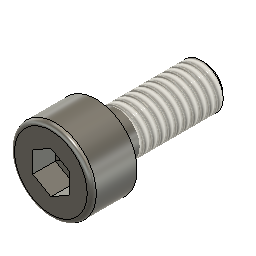
Spacemouse_3D_model (Autodesk Fusion 360 archive; units mm, degrees)
design "Broached Hexagon Socket Head Cap Screw ASME B18.3.1M - M2.5x0.45 x 6 Steel Grade 2 Plain"
description: Broached Hexagon Socket Head Cap Screw ASME B18.3.1M - M2.5x0.45 x 6
part number: BSHCS ASME B18.3.1M - M2.5x0.45 x 6 Steel Grade 2 Plain
Autodesk Fusion 360 part; units mm, degrees
sketch "Sketch1" plane through (0, 0, 0) normal (0, 1, 0) x (1, 0, 0)
  line L0 (-1.25, 0) -> (-1.25, 6)
  line L1 (-1.25, 6) -> (0, 6)
  line L2 (0, 6) -> (0, -2.5)
  line L3 (-1.25, 0) -> (-2.25, 0)
  line L4 (-2.25, 0) -> (-2.25, -2.5)
  line L5 (-2.25, -2.5) -> (0, -2.5)
  dimension "d101" = 6
  dimension "d102" = 2.5
  dimension "d109" = 4.5
  dimension "d110" = 2.5
  constraint perpendicular L0 L1
  constraint collinear origin L1.end L2.end
  constraint perpendicular L0 L3
  constraint coincident origin L3
  constraint vertical L2
  constraint coincident L2 L5.end
  constraint perpendicular L2 L5
  measures "d101" distance of origin L1
  measures "d102" distance of L3.end L5
revolve "Revolve1" add sketch "Sketch1" angle 360 about axis through (0, 0, -6) along (0, 0, 1)
ref_plane "WorkPlane1" through (0, 0, 2.5) normal (0, 0, 1) x (1, 0, 0)
sketch "Sketch6" plane through (0, 0, 2.5) normal (0, 0, 1) x (1, 0, 0)
  line L0 (0, -1.1547) -> (1, -0.5774)
  line L1 (1, -0.5774) -> (1, 0.5774)
  line L2 (1, 0.5774) -> (0, 1.1547)
  line L3 (0, 1.1547) -> (-1, 0.5774)
  line L4 (-1, 0.5774) -> (-1, -0.5774)
  line L5 (-1, -0.5774) -> (0, -1.1547)
  dimension "d111" = 2
  constraint vertical L1
  measures "d111" distance of L1 L4
extrude "Extrude1" cut sketch "Sketch6" against normal blind 1.25
extrude "Extrude2" cut 1 faces at (-0.3333, -0.1925, 1.25) along direction (0, 0, -1) blind 1.25 draft -85
thread "Thread3" "ANSI Metric M Profile 2.5 M2.5x0.45 M2.5x0.45 4g6g" major diameter 2.43 minor diameter 1.9295 pitch 0.45 angle 60 resizes the face on face at (-1.2438, 0.1245, -4) from (0, 0, -1.1761) to (0, 0, -6)
fillet "Fillet4" radius 0.25 1 edges at (-2.0977, 0.8136, 2.5)
sketch "Sketch7" plane through (0, 0, 0) normal (0, 1, 0) x (1, 0, 0)
  line L0 (-1.275, 6) -> (-1.275, 5.7239)
  line L1 (-1.275, 5.7239) -> (-0.9739, 6)
  line L2 (0, 6) -> (0, -2.5)
  line L3 (-1.275, 6) -> (0, 6)
  dimension "d104" = 0.9739
  dimension "d105" = 1.275
  dimension "d106" = 0.2761
  constraint coincident L2.start L3.end
  constraint perpendicular L2 L3
  constraint coincident L1.end L3
  constraint perpendicular L0 L3
  measures "d104" distance of L1.end L2
  measures "d105" distance of L0 L2.start
  measures "d106" distance of L0.end L3
revolve "Revolve3" cut sketch "Sketch7" angle 360 about axis through (0, 0, 1.75) along (0, 0, 1)
equation "adsk_nomlen = 6.000 mm"
equation "adsk_headh = 2.500 mm"
equation "adsk_headdia = 4.500 mm"
equation "adsk_nomdia = 2.500 mm"
equation "adsk_philwidth = 2.000 mm"
equation "d31 = -adsk_phildepth"
equation "adsk_phildepth = 1.250 mm"
equation "d71 = adsk_headh"
equation "d76 = -adsk_phildepth"
equation "adsk_thrlen = 4.8239475 mm"
equation "d86 = adsk_nomdia * 0.1"
equation "adsk_startlen = 0.2760525 mm"
equation "adsk_endpointdia = 1.947895 mm"
equation "d101 = adsk_nomlen"
equation "d102 = adsk_headh"
equation "d104 = adsk_endpointdia / 2"
equation "d105 = adsk_nomdia * 0.51"
equation "d106 = adsk_startlen"
equation "d108 = min(adsk_thrlen; adsk_nomlen - 0.001 mm)"
equation "d109 = adsk_headdia"
equation "d110 = adsk_nomdia"
equation "d111 = adsk_philwidth"

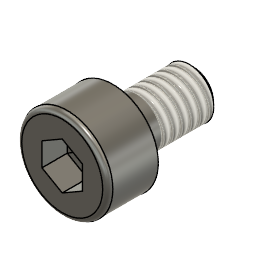
design "Vis percée à tête à six pans creux ASME B18.3.1M - M2.5x0.45 x 4 Acier de classe 2 Standard"
description: Vis percée à tête à six pans creux ASME B18.3.1M - M2.5x0.45 x 4
part number: BSHCS ASME B18.3.1M - M2.5x0.45 x 4 Acier de classe 2 Standard
Autodesk Fusion 360 part; units mm, degrees
sketch "Sketch1" plane through (0, 0, 0) normal (0, 1, 0) x (1, 0, 0)
  line L0 (-1.25, 0) -> (-1.25, 4)
  line L1 (-1.25, 4) -> (0, 4)
  line L2 (0, 4) -> (0, -2.5)
  line L3 (-1.25, 0) -> (-2.25, 0)
  line L4 (-2.25, 0) -> (-2.25, -2.5)
  line L5 (-2.25, -2.5) -> (0, -2.5)
  dimension "d101" = 4
  dimension "d102" = 2.5
  dimension "d109" = 4.5
  dimension "d110" = 2.5
  constraint perpendicular L0 L1
  constraint collinear origin L1.end L2.end
  constraint perpendicular L0 L3
  constraint coincident origin L3
  constraint vertical L2
  constraint coincident L2 L5.end
  constraint perpendicular L2 L5
  measures "d101" distance of origin L1
  measures "d102" distance of L3.end L5
revolve "Revolve1" add sketch "Sketch1" angle 360 about axis through (0, 0, -4) along (0, 0, 1)
ref_plane "WorkPlane1" through (0, 0, 2.5) normal (0, 0, 1) x (1, 0, 0)
sketch "Sketch6" plane through (0, 0, 2.5) normal (0, 0, 1) x (1, 0, 0)
  line L0 (0, -1.1547) -> (1, -0.5774)
  line L1 (1, -0.5774) -> (1, 0.5774)
  line L2 (1, 0.5774) -> (0, 1.1547)
  line L3 (0, 1.1547) -> (-1, 0.5774)
  line L4 (-1, 0.5774) -> (-1, -0.5774)
  line L5 (-1, -0.5774) -> (0, -1.1547)
  dimension "d111" = 2
  constraint vertical L1
  measures "d111" distance of L1 L4
extrude "Extrude1" cut sketch "Sketch6" against normal blind 1.25
extrude "Extrude2" cut 1 faces at (-0.3333, -0.1925, 1.25) along direction (0, 0, -1) blind 1.25 draft -85
thread "Thread3" "ANSI Metric M Profile 2.5 M2.5x0.45 M2.5x0.45 4g6g" major diameter 2.43 minor diameter 1.9295 pitch 0.45 angle 60 resizes the face on face at (-1.2484, 0.0623, -2.6667) from (0, 0, -1.1761) to (0, 0, -4)
fillet "Fillet4" radius 0.25 1 edges at (-2.0977, 0.8136, 2.5)
sketch "Sketch7" plane through (0, 0, 0) normal (0, 1, 0) x (1, 0, 0)
  line L0 (-1.275, 4) -> (-1.275, 3.7239)
  line L1 (-1.275, 3.7239) -> (-0.9739, 4)
  line L2 (0, 4) -> (0, -2.5)
  line L3 (-1.275, 4) -> (0, 4)
  dimension "d104" = 0.9739
  dimension "d105" = 1.275
  dimension "d106" = 0.2761
  constraint coincident L2.start L3.end
  constraint perpendicular L2 L3
  constraint coincident L1.end L3
  constraint perpendicular L0 L3
  measures "d104" distance of L1.end L2
  measures "d105" distance of L0 L2.start
  measures "d106" distance of L0.end L3
revolve "Revolve3" cut sketch "Sketch7" angle 360 about axis through (0, 0, 1.75) along (0, 0, 1)
equation "adsk_nomlen = 4.000 mm"
equation "adsk_headh = 2.500 mm"
equation "adsk_headdia = 4.500 mm"
equation "adsk_nomdia = 2.500 mm"
equation "adsk_philwidth = 2.000 mm"
equation "d31 = -adsk_phildepth"
equation "adsk_phildepth = 1.250 mm"
equation "d71 = adsk_headh"
equation "d76 = -adsk_phildepth"
equation "adsk_thrlen = 2.8239475 mm"
equation "d86 = adsk_nomdia * 0.1"
equation "adsk_startlen = 0.2760525 mm"
equation "adsk_endpointdia = 1.947895 mm"
equation "d101 = adsk_nomlen"
equation "d102 = adsk_headh"
equation "d104 = adsk_endpointdia / 2"
equation "d105 = adsk_nomdia * 0.51"
equation "d106 = adsk_startlen"
equation "d108 = min(adsk_thrlen; adsk_nomlen - 0.001 mm)"
equation "d109 = adsk_headdia"
equation "d110 = adsk_nomdia"
equation "d111 = adsk_philwidth"

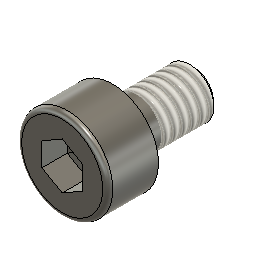
design "Broached Hexagon Socket Head Cap Screw ASME B18.3.1M - M2.5x0.45 x 4 Steel Grade 2 Plain"
description: Broached Hexagon Socket Head Cap Screw ASME B18.3.1M - M2.5x0.45 x 4
part number: BSHCS ASME B18.3.1M - M2.5x0.45 x 4 Steel Grade 2 Plain
Autodesk Fusion 360 part; units mm, degrees
sketch "Sketch1" plane through (0, 0, 0) normal (0, 1, 0) x (1, 0, 0)
  line L0 (-1.25, 0) -> (-1.25, 4)
  line L1 (-1.25, 4) -> (0, 4)
  line L2 (0, 4) -> (0, -2.5)
  line L3 (-1.25, 0) -> (-2.25, 0)
  line L4 (-2.25, 0) -> (-2.25, -2.5)
  line L5 (-2.25, -2.5) -> (0, -2.5)
  dimension "d101" = 4
  dimension "d102" = 2.5
  dimension "d109" = 4.5
  dimension "d110" = 2.5
  constraint perpendicular L0 L1
  constraint collinear origin L1.end L2.end
  constraint perpendicular L0 L3
  constraint coincident origin L3
  constraint vertical L2
  constraint coincident L2 L5.end
  constraint perpendicular L2 L5
  measures "d101" distance of origin L1
  measures "d102" distance of L3.end L5
revolve "Revolve1" add sketch "Sketch1" angle 360 about axis through (0, 0, -4) along (0, 0, 1)
ref_plane "WorkPlane1" through (0, 0, 2.5) normal (0, 0, 1) x (1, 0, 0)
sketch "Sketch6" plane through (0, 0, 2.5) normal (0, 0, 1) x (1, 0, 0)
  line L0 (0, -1.1547) -> (1, -0.5774)
  line L1 (1, -0.5774) -> (1, 0.5774)
  line L2 (1, 0.5774) -> (0, 1.1547)
  line L3 (0, 1.1547) -> (-1, 0.5774)
  line L4 (-1, 0.5774) -> (-1, -0.5774)
  line L5 (-1, -0.5774) -> (0, -1.1547)
  dimension "d111" = 2
  constraint vertical L1
  measures "d111" distance of L1 L4
extrude "Extrude1" cut sketch "Sketch6" against normal blind 1.25
extrude "Extrude2" cut 1 faces at (-0.3333, -0.1925, 1.25) along direction (0, 0, -1) blind 1.25 draft -85
thread "Thread3" "ANSI Metric M Profile 2.5 M2.5x0.45 M2.5x0.45 4g6g" major diameter 2.43 minor diameter 1.9295 pitch 0.45 angle 60 resizes the face on face at (-1.2484, 0.0623, -2.6667) from (0, 0, -1.1761) to (0, 0, -4)
fillet "Fillet4" radius 0.25 1 edges at (-2.0977, 0.8136, 2.5)
sketch "Sketch7" plane through (0, 0, 0) normal (0, 1, 0) x (1, 0, 0)
  line L0 (-1.275, 4) -> (-1.275, 3.7239)
  line L1 (-1.275, 3.7239) -> (-0.9739, 4)
  line L2 (0, 4) -> (0, -2.5)
  line L3 (-1.275, 4) -> (0, 4)
  dimension "d104" = 0.9739
  dimension "d105" = 1.275
  dimension "d106" = 0.2761
  constraint coincident L2.start L3.end
  constraint perpendicular L2 L3
  constraint coincident L1.end L3
  constraint perpendicular L0 L3
  measures "d104" distance of L1.end L2
  measures "d105" distance of L0 L2.start
  measures "d106" distance of L0.end L3
revolve "Revolve3" cut sketch "Sketch7" angle 360 about axis through (0, 0, 1.75) along (0, 0, 1)
equation "adsk_nomlen = 4.000 mm"
equation "adsk_headh = 2.500 mm"
equation "adsk_headdia = 4.500 mm"
equation "adsk_nomdia = 2.500 mm"
equation "adsk_philwidth = 2.000 mm"
equation "d31 = -adsk_phildepth"
equation "adsk_phildepth = 1.250 mm"
equation "d71 = adsk_headh"
equation "d76 = -adsk_phildepth"
equation "adsk_thrlen = 2.8239475 mm"
equation "d86 = adsk_nomdia * 0.1"
equation "adsk_startlen = 0.2760525 mm"
equation "adsk_endpointdia = 1.947895 mm"
equation "d101 = adsk_nomlen"
equation "d102 = adsk_headh"
equation "d104 = adsk_endpointdia / 2"
equation "d105 = adsk_nomdia * 0.51"
equation "d106 = adsk_startlen"
equation "d108 = min(adsk_thrlen; adsk_nomlen - 0.001 mm)"
equation "d109 = adsk_headdia"
equation "d110 = adsk_nomdia"
equation "d111 = adsk_philwidth"

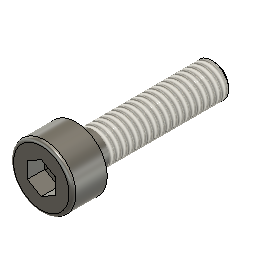
design "Broached Hexagon Socket Head Cap Screw ASME B18.3.1M - M2.5x0.45 x 10 Steel Grade 2 Plain"
description: Broached Hexagon Socket Head Cap Screw ASME B18.3.1M - M2.5x0.45 x 10
part number: BSHCS ASME B18.3.1M - M2.5x0.45 x 10 Steel Grade 2 Plain
Autodesk Fusion 360 part; units mm, degrees
sketch "Sketch1" plane through (0, 0, 0) normal (0, 1, 0) x (1, 0, 0)
  line L0 (-1.25, 0) -> (-1.25, 10)
  line L1 (-1.25, 10) -> (0, 10)
  line L2 (0, 10) -> (0, -2.5)
  line L3 (-1.25, 0) -> (-2.25, 0)
  line L4 (-2.25, 0) -> (-2.25, -2.5)
  line L5 (-2.25, -2.5) -> (0, -2.5)
  dimension "d101" = 10
  dimension "d102" = 2.5
  dimension "d109" = 4.5
  dimension "d110" = 2.5
  constraint perpendicular L0 L1
  constraint collinear origin L1.end L2.end
  constraint perpendicular L0 L3
  constraint coincident origin L3
  constraint vertical L2
  constraint coincident L2 L5.end
  constraint perpendicular L2 L5
  measures "d101" distance of origin L1
  measures "d102" distance of L3.end L5
revolve "Revolve1" add sketch "Sketch1" angle 360 about axis through (0, 0, -10) along (0, 0, 1)
ref_plane "WorkPlane1" through (0, 0, 2.5) normal (0, 0, 1) x (1, 0, 0)
sketch "Sketch6" plane through (0, 0, 2.5) normal (0, 0, 1) x (1, 0, 0)
  line L0 (0, -1.1547) -> (1, -0.5774)
  line L1 (1, -0.5774) -> (1, 0.5774)
  line L2 (1, 0.5774) -> (0, 1.1547)
  line L3 (0, 1.1547) -> (-1, 0.5774)
  line L4 (-1, 0.5774) -> (-1, -0.5774)
  line L5 (-1, -0.5774) -> (0, -1.1547)
  dimension "d111" = 2
  constraint vertical L1
  measures "d111" distance of L1 L4
extrude "Extrude1" cut sketch "Sketch6" against normal blind 1.25
extrude "Extrude2" cut 1 faces at (-0.3333, -0.1925, 1.25) along direction (0, 0, -1) blind 1.25 draft -85
thread "Thread3" "ANSI Metric M Profile 2.5 M2.5x0.45 M2.5x0.45 4g6g" major diameter 2.43 minor diameter 1.9295 pitch 0.45 angle 60 resizes the face on face at (-1.2438, 0.1245, -6.6667) from (0, 0, -1.1761) to (0, 0, -10)
fillet "Fillet4" radius 0.25 1 edges at (-2.0977, 0.8136, 2.5)
sketch "Sketch7" plane through (0, 0, 0) normal (0, 1, 0) x (1, 0, 0)
  line L0 (-1.275, 10) -> (-1.275, 9.7239)
  line L1 (-1.275, 9.7239) -> (-0.9739, 10)
  line L2 (0, 10) -> (0, -2.5)
  line L3 (-1.275, 10) -> (0, 10)
  dimension "d104" = 0.9739
  dimension "d105" = 1.275
  dimension "d106" = 0.2761
  constraint coincident L2.start L3.end
  constraint perpendicular L2 L3
  constraint coincident L1.end L3
  constraint perpendicular L0 L3
  measures "d104" distance of L1.end L2
  measures "d105" distance of L0 L2.start
  measures "d106" distance of L0.end L3
revolve "Revolve3" cut sketch "Sketch7" angle 360 about axis through (0, 0, 1.75) along (0, 0, 1)
equation "adsk_nomlen = 10.000 mm"
equation "adsk_headh = 2.500 mm"
equation "adsk_headdia = 4.500 mm"
equation "adsk_nomdia = 2.500 mm"
equation "adsk_philwidth = 2.000 mm"
equation "d31 = -adsk_phildepth"
equation "adsk_phildepth = 1.250 mm"
equation "d71 = adsk_headh"
equation "d76 = -adsk_phildepth"
equation "adsk_thrlen = 8.8239475 mm"
equation "d86 = adsk_nomdia * 0.1"
equation "adsk_startlen = 0.2760525 mm"
equation "adsk_endpointdia = 1.947895 mm"
equation "d101 = adsk_nomlen"
equation "d102 = adsk_headh"
equation "d104 = adsk_endpointdia / 2"
equation "d105 = adsk_nomdia * 0.51"
equation "d106 = adsk_startlen"
equation "d108 = min(adsk_thrlen; adsk_nomlen - 0.001 mm)"
equation "d109 = adsk_headdia"
equation "d110 = adsk_nomdia"
equation "d111 = adsk_philwidth"
